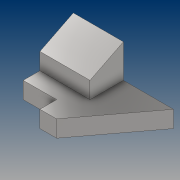
# Autodesk Inventor part: 43
Saved by Autodesk Inventor 2020.2 (Build 242310000, 310)
## iProperties
Created: 2020-09-17
Part Number: 43
Material: 鋼、碳鋼
Document SubType Name: Modeling
Designer: user
Density: 7.85 g/cm^3
Appearance: 半拋光
Mass: 196.25 g
Surface Area: 65.7082 cm^2
Volume: 25 cm^3
Author: user
Autodesk Inventor part; units mm, degrees
ref_plane "YZ Plane" through (0, 0, 0) normal (1, 0, 0) x (0, 1, 0)
ref_plane "XZ Plane" through (0, 0, 0) normal (0, 1, 0) x (-1, 0, 0)
ref_plane "XY Plane" through (0, 0, 0) normal (0, 0, 1) x (1, 0, 0)
sketch "草圖1" plane through (0, 0, 0) normal (0, 1, 0) x (-1, 0, 0)
  line L0 (0, 0) -> (0, 30)
  line L1 (0, 30) -> (-20, 30)
  line L2 (-20, 30) -> (-20, 40)
  line L3 (-20, 40) -> (-30, 40)
  line L4 (-30, 40) -> (-60, 0)
  line L5 (-60, 0) -> (0, 0)
  dimension "d0" = 30
  dimension "d1" = 10
  dimension "d2" = 20
  dimension "d3" = 60
  dimension "d4" = 10
  constraints: 12 end point, 3 perpendicular, 1 parallel, 1 vertical
  measures "d0" distance of L0.start L0.end
  measures "d1" distance of L1.end L2.end
  measures "d2" distance of L0.end L1.end
  measures "d3" distance of L4.end L0.start
  measures "d4" distance of L2.end L3.end
extrude "擠出1" add sketch "草圖1" along normal blind 10
sketch "草圖2" plane through (0, 10, 0) normal (0, 1, 0) x (1, 0, 0)
  line L0 (30, -40) -> (20, -40) projected
  line L1 (20, -40) -> (20, -30) projected
  line L2 (20, -30) -> (0, -30) projected
  line L3 (0, -30) -> (0, 0) projected
  line L4 (0, 0) -> (60, 0) projected
  line L5 (60, 0) -> (30, -40) projected
  line L6 (60, 0) -> (0, 0) projected
  line L7 (0, 0) -> (30, 0)
  line L8 (30, 0) -> (30, -20)
  line L9 (30, -20) -> (0, -20)
  line L10 (0, -20) -> (0, 0)
  dimension "d7" = 30
  dimension "d8" = 20
  constraints: 8 end point, 2 parallel, 1 horizontal, 1 perpendicular
  measures "d7" distance of L8.end L9.end
  measures "d8" distance of L7.end L8.end
extrude "擠出2" add sketch "草圖2" along normal blind 20 contours L8 L9 L3 L4
sketch "草圖3" plane through (30, 10, 20) normal (1, 0, 0) x (0, 0, -1)
  line L0 (0, 0) -> (0, 20) projected
  line L1 (0, 20) -> (20, 20) projected
  line L2 (20, 20) -> (20, 0) projected
  line L3 (0, 0) -> (20, 0) projected
  line L4 (-20, 0) -> (0, 0) projected
  line L5 (-20, -10) -> (-20, 0) projected
  line L6 (20, -10) -> (-20, -10) projected
  line L7 (20, 0) -> (20, -10) projected
  line L8 (0, 0) -> (0, 20) projected
  line L9 (0, 10) -> (20, 20)
  line L10 (20, 0) -> (20, 20) projected
  dimension "d11" = 10
  constraints: 2 end point, 1 midpoint
  measures "d11" distance from line of L1 L9.start
extrude "擠出3" cut sketch "草圖3" against normal through all contours L0 L1 L9
